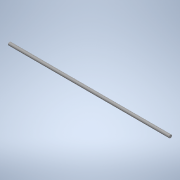
# Autodesk Inventor part: 8x435axis
Saved by Autodesk Inventor 2020.2 (Build 242310000, 310)
## iProperties
CustomPartVersion: 1
Created: 2017-10-26
Part Number: 8x435axis
Material: Steel
Document SubType Name: Modeling
Designer: wojte
Density: 1 g/cm^3
Appearance: Steel
Author: wojte
Autodesk Inventor part; units mm, degrees
ref_plane "Płaszczyzna początkowa" through (0, 0, 0) normal (1, 0, 0) x (0, 1, 0)
ref_plane "XZ Plane" through (0, 0, 0) normal (0, 1, 0) x (-1, 0, 0)
ref_plane "XY Plane" through (0, 0, 0) normal (0, 0, 1) x (1, 0, 0)
sketch "Szkic główny" plane through (0, 0, 0) normal (0, 0, 1) x (1, 0, 0)
  line L0 (0, 0) -> (433.5, 0)
  line L1 (0, 0) -> (0, 4)
  line L2 (433.5, 4) -> (433.5, 0)
  line L3 (0, 4) -> (433.5, 4)
  dimension "d3" = 8
  constraints: 8 end point, 3 horizontal, 2 vertical
  measures "d3" diameter of L3 L0
revolve "Obrót1" add sketch "Szkic główny" angle 360 about axis through (0, 0, 0) along (1, 0, 0)
